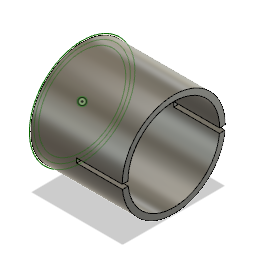
WormObserver_V2_objective_adapter (Autodesk Fusion 360 design; units mm, degrees)
Autodesk Fusion 360 part; units mm, degrees
note: some values were not read from the file. Set by a fixed rule: which sketch regions a step uses.
sketch "Sketch1" plane through (0, 0, 0) normal (1, 0, 0) x (0, 0, -1)
  circle A0 centre (0, 0) radius 23
  circle A1 centre (0, 0) radius 19
  circle A2 centre (0, 0) radius 21
  dimension "d1" = 46
  dimension "d2" = 4
  dimension "d3" = 2
  measures "d1" diameter of A0
  measures "d2" distance of A0 A1
  measures "d3" distance of A1 A2
extrude "Extrude5" add sketch "Sketch1" along normal blind 40 contours A0
extrude "Extrude6" add sketch "Sketch1" along normal blind 5 contours A2
move_face "OffsetFaces2" offset -0.5 1 faces at (26.6667, -1.1465, -22.9714)
move_face "OffsetFaces3" offset 1 1 faces at (28.3333, 2.0909, -20.8956)
move_face "OffsetFaces4" offset 2 1 faces at (1.6667, 0.9471, -18.9764)
box "BoxPrimitive1" cut length 2 width 4.5 height -20 placed x (0, 1, 0) y (0, 0, 1) z (1, 0, 0) at (40, -2.0003, -22.9945)
box "BoxPrimitive2" cut length 2 width 4 height -20 placed x (0, -1, 0) y (0, 0, -1) z (1, 0, 0) at (40, -0.0265, 23)
extrude "Extrude3" [suppressed]
extrude "Extrude2" [suppressed]
extrude "Extrude1" [suppressed]
other "CylinderPrimitive1"
move_face "OffsetFaces1" [suppressed]
extrude "Extrude4" [suppressed]
